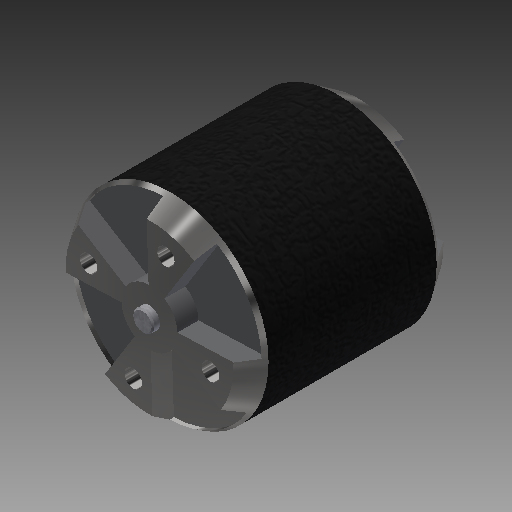
# Autodesk Inventor part: 2830-1100 KV MOTOR
Saved by Autodesk Inventor 2019 (Build 230136000, 136)
## iProperties
Created: 2014-01-01
Part Number: 2830-1100 KV MOTOR
Document SubType Name: Modeling
Designer: user
Density: 1 g/cm^3
Material: Generic
Appearance: Steel - Polished
Author: user
Autodesk Inventor part; units mm, degrees
ref_plane "XZ Plane" through (0, 0, 0) normal (0, 1, 0) x (-1, 0, 0)
ref_plane "XY Plane" through (0, 0, 0) normal (0, 0, 1) x (1, 0, 0)
sketch "Sketch1" plane through (0, 0, 0) normal (0, 0, 1) x (1, 0, 0)
  circle A0 centre (0, 0) radius 14
  dimension "d0" = 28
  constraints: 1 centre point, 1 coincident
  measures "d0" diameter of A0
extrude "Extrusion1" add sketch "Sketch1" along normal blind 30
chamfer "Chamfer1" distance 2 distance2 3 1 edges at (-14, 0, 0) measured on face at (0.5625, 1.5565, 0)
chamfer "Chamfer2" distance 2 distance2 3 1 edges at (-14, 0, 30) measured on face at (0.5625, 1.5565, 30)
sketch "Sketch2" plane through (0, 0, 0) normal (0, 0, -1) x (-1, 0, 0)
  circle A0 centre (0, 0) radius 12 projected
  circle A1 centre (0, 0) radius 4
  dimension "d9" = 8
  constraints: 1 centre point, 1 coincident
  measures "d9" diameter of A1
extrude "Extrusion2" add sketch "Sketch2" along normal blind 1.4 contours A1
sketch "Sketch3" plane through (0, 0, 0) normal (0, 0, -1) x (-1, 0, 0)
  circle A0 centre (0, 0) radius 4 projected
  circle A1 centre (0, 0) radius 12 projected
  line L0 (0, 0) -> (0, -20.1603) construction
  line L1 (0, 0) -> (8.5074, -16)
  line L2 (8.5074, -16) -> (0, -16)
  line L3 (0, 0) -> (-8.5074, -16)
  line L4 (-8.5074, -16) -> (0, -16)
  dimension "d12" = 28
  dimension "d13" = 16
  constraints: 10 end point, 1 perpendicular, 1 point on line, 1 symmetric about line, 1 vertical
  measures "d12" angle of L0 L1
  measures "d13" distance from line of A0.centre L2
extrude "Extrusion3" cut sketch "Sketch3" against normal blind 2.4 contours L3 L1 A0 | A0 L1 A1 L3 | A1 L1 L2 L4 L3 picked at (0.9485, -2.471) picked at (3.4716, -8.5902)
pattern_circular "Circular Pattern1" count 3 over 360 about axis through (0, 0, 0) along (0, 0, -1) of "Extrusion3"
sketch "Sketch4" plane through (0, 0, 0) normal (0, 0, -1) x (-1, 0, 0)
  arc A0 (2.1197, 3.3922) -> (-2.1197, 3.3922) centre (0, 0) ccw projected
  arc A1 (6.359, 10.1766) -> (-6.359, 10.1766) centre (0, 0) ccw projected
  line L0 (0, 0) -> (0, 17.8727) construction
  point P0 (0, 8)
  dimension "d19" = 8
  constraints: 2 end point, 1 point on line, 1 vertical
  measures "d19" distance of A0.centre point (0, 8)
hole "Hole1" at (0, 8, 0) direction (0, 0, 1) diameter 2.013 depth 4 tip angle 118 thread size "M2.5x0.45" class "6H" standard "ANSI Metric M Profile"
pattern_circular "Circular Pattern2" count 3 over 360 about axis through (0, 0, 0) along (0, 0, -1) of "Hole1"
sketch "Sketch6" plane through (0, 0, 0) normal (0, 0, 1) x (1, 0, 0)
  arc A0 (-1.8779, -3.5318) -> (1.8779, -3.5318) centre (0, 0) ccw projected
  line L0 (1.8779, -3.5318) -> (0, 0) projected
  line L1 (0, 0) -> (-1.8779, -3.5318) projected
  arc A1 (-2.1197, 3.3922) -> (-3.9976, 0.1396) centre (0, 0) ccw projected
  line L2 (-3.9976, 0.1396) -> (0, 0) projected
  line L3 (0, 0) -> (-2.1197, 3.3922) projected
  arc A2 (3.9976, 0.1396) -> (2.1197, 3.3922) centre (0, 0) ccw projected
  line L4 (2.1197, 3.3922) -> (0, 0) projected
  line L5 (0, 0) -> (3.9976, 0.1396) projected
extrude "Extrusion4" add sketch "Sketch6" along normal up to next
sketch "Sketch7" plane through (0, 0, 30) normal (0, 0, 1) x (1, 0, 0)
  arc A0 (3.9976, 0.1396) -> (2.1197, 3.3922) centre (0, 0) ccw projected
  line L0 (2.1197, 3.3922) -> (7.2069, 11.5335) projected
  arc A1 (13.5917, 0.4746) -> (7.2069, 11.5335) centre (0, 0) ccw projected
  line L1 (13.5917, 0.4746) -> (3.9976, 0.1396) projected
extrude "Extrusion5" cut sketch "Sketch7" against normal blind 3
pattern_circular "Circular Pattern3" count 4 over 360 about axis through (0, 0, 0) along (0, 0, 1) of "Extrusion5"
sketch "Sketch8" plane through (0, 0, 30) normal (0, 0, 1) x (1, 0, 0)
  arc A0 (-10.1766, 6.359) -> (-11.9927, -0.4188) centre (0, 0) ccw projected
  circle A1 centre (0, 0) radius 1.5
  dimension "d37" = 3
  constraints: 1 centre point, 1 coincident
  measures "d37" diameter of A1
extrude "Extrusion6" add sketch "Sketch8" along normal blind 1
chamfer "Chamfer3" distance 0.2 angle 45 1 edges at (-1.5, 0, 31)
sketch "Sketch9" plane through (0, 0, 30) normal (0, 0, 1) x (1, 0, 0)
  circle A0 centre (0, 0) radius 1.5 projected
  arc A1 (-10.1766, 6.359) -> (-11.9927, -0.4188) centre (0, 0) ccw projected
  arc A2 (-6.359, -10.1766) -> (0.4188, -11.9927) centre (0, 0) ccw projected
  line L0 (0, 0) -> (-11.5911, 3.1058) construction
  circle A3 centre (-8.6933, 2.3294) radius 1.25
  dimension "d43" = 2.5
  dimension "d44" = 9
  constraints: 2 end point, 1 centre point, 1 point on circle, 1 point on line
  measures "d43" diameter of A3
  measures "d44" distance of A0.centre A3.centre
extrude "Extrusion7" cut sketch "Sketch9" against normal blind 5 contours A3
pattern_circular "Circular Pattern4" count 4 over 360 about axis through (0, 0, 30) along (0, 0, 1) of "Extrusion7"
ref_plane "Work Plane1" through (14, 0, 0) normal (1, 0, 0) x (0, 1, 0)
sketch "Sketch10" plane through (14, 0, 0) normal (1, 0, 0) x (0, 1, 0)
  line L0 (18.3657, 31.0207) -> (17.8778, 30.841) construction
  line L1 (14, 27) -> (-14, 27) construction
  line L2 (-14, 3) -> (14, 3) construction
  line L3 (-7.4484, 3) -> (-7.4484, 27) construction
  line L4 (-7.4484, 27) -> (7.4484, 27) construction
  line L5 (7.4484, 27) -> (7.4484, 3) construction
  line L6 (7.4484, 3) -> (-7.4484, 3) construction
  point P0 (0, 3)
  point P1 (0, 27)
  constraints: 4 midpoint, 2 end point, 2 other
decal "Decal1"
body "Solid1"
